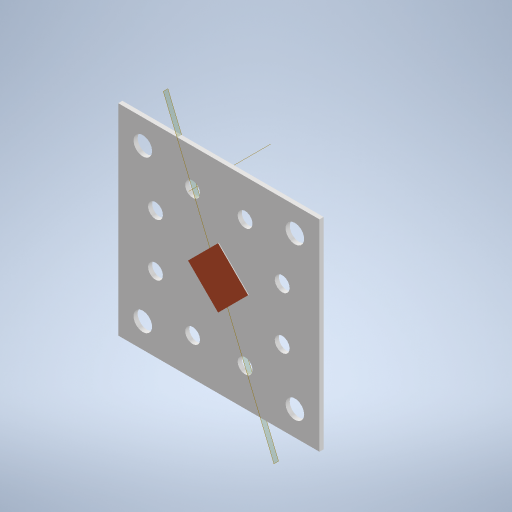
# Autodesk Inventor part: PCB
Saved by Autodesk Inventor 2023.1 (Build 271208000, 208)
## iProperties
Company: Aalto University / OtaNano
Created: 2023-02-06
Part Number: PCB
Material: Generic
Document SubType Name: Modeling
Designer: Joel Salminen
Density: 1 g/cm^3
Appearance: Default
Mass: 0.386419 g
Surface Area: 14.7697 cm^2
Volume: 0.386419 cm^3
Author: Joel Salminen
Autodesk Inventor part; units mm, degrees
ref_plane "YZ Plane" through (0, 0, 0) normal (1, 0, 0) x (0, 1, 0)
ref_plane "XZ Plane" through (0, 0, 0) normal (0, 1, 0) x (-1, 0, 0)
ref_plane "XY Plane" through (0, 0, 0) normal (0, 0, 1) x (1, 0, 0)
sketch "Sketch1" plane through (0, 0, 0) normal (0, 0, 1) x (1, 0, 0)
  line L0 (13.5, -13.5) -> (-13.5, -13.5)
  line L1 (-13.5, -13.5) -> (-13.5, 13.5)
  line L2 (-13.5, 13.5) -> (13.5, 13.5)
  line L3 (13.5, 13.5) -> (13.5, -13.5)
  line L4 (13.5, -13.5) -> (-13.5, 13.5) construction
  line L5 (-13.5, -13.5) -> (13.5, 13.5) construction
  point P0 (0, 0)
  dimension "d0" = 27
  constraints: 12 end point, 2 midpoint, 2 parallel, 2 perpendicular, 1 horizontal
  measures "d0" distance of L1.end L2.end
extrude "Extrusion1" add sketch "Sketch1" along normal mid plane 0.56
sketch "Sketch2" plane through (0, 0, 0.28) normal (0, 0, 1) x (1, 0, 0)
  line L0 (-13.5, -13.5) -> (13.5, -13.5) projected
  line L1 (13.5, -13.5) -> (13.5, 13.5) projected
  line L2 (0, 0) -> (0, -13.5)
  line L3 (0, 0) -> (13.5, 0)
  point P0 (10.2, -10.2)
  dimension "d3" = 20.4
  dimension "d4" = 20.4
  constraints: 4 end point, 2 midpoint
  measures "d3" diameter of point (10.2, -10.2) L2
  measures "d4" diameter of point (10.2, -10.2) L3
hole "Hole1" at (10.2, -10.2, 0.28) direction (0, 0, -1) diameter 2.5 end through all
pattern_circular "Circular Pattern1" count 4 over 360 about axis through (0, 0, -10) along (0, 0, 1) of "Hole1"
sketch "Sketch3" plane through (0, 0, 0.28) normal (0, 0, 1) x (1, 0, 0)
  circle A0 centre (-3.52, 8.5) radius 1
  point P0 (0, 0)
  dimension "d15" = 2
  dimension "d16" = 3.52
  dimension "d17" = 8.5
  constraints: 1 centre point
  measures "d15" diameter of A0
  measures "d16" horizontal distance of point (0, 0) A0.centre
  measures "d17" vertical distance of point (0, 0) A0.centre
extrude "Extrusion2" cut sketch "Sketch3" against normal through all
mirror "Mirror1" about plane through (0, 0, 0) normal (1, 0, 0) of "Extrusion2"
pattern_circular "Circular Pattern2" count 4 over 360 about axis through (0, 0, -10) along (0, 0, 1) of "Extrusion2", "Mirror1"
ref_plane "Work Plane1" through (-3.52, 8.5, 0.28) normal (-0.9239, -0.3826, 0) x (0, 0, -1)
sketch "Sketch4" plane through (0, 0, 0.28) normal (0, 0, 1) x (1, 0, 0)
  line L0 (-4.0305, 0) -> (0, 4.0305)
  line L1 (0, 4.0305) -> (4.0305, 0)
  line L2 (4.0305, 0) -> (0, -4.0305)
  line L3 (0, -4.0305) -> (-4.0305, 0)
  line L4 (0, 4.0305) -> (0, -4.0305) construction
  line L5 (-4.0305, 0) -> (4.0305, 0) construction
  point P0 (0, 0)
  point P1 (0, 0)
  dimension "d23" = 5.7
  constraints: 12 end point, 2 midpoint, 1 coincident, 1 horizontal, 1 perpendicular, 1 vertical
  measures "d23" distance of L1.end L2.end
extrude "Extrusion3" add sketch "Sketch4" along normal blind 0.1
equation "\"d4\" = d3"
body "Solid1"
